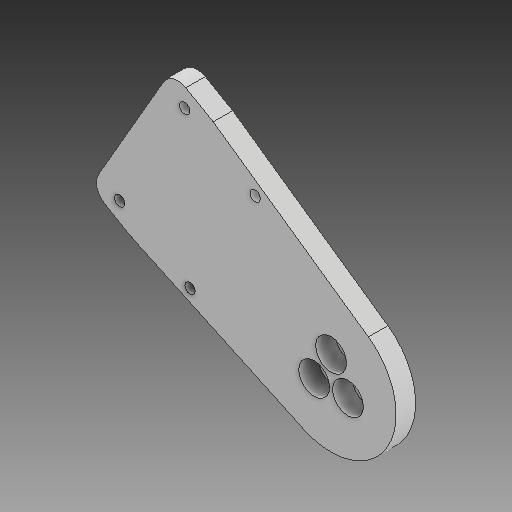
# Autodesk Inventor part: Кронштейн_разлив
Saved by Autodesk Inventor 2022 (Build 260153000, 153)
## iProperties
Created: 2025-01-18
Part Number: Кронштейн_разлив
Material: Типовые
Document SubType Name: Modeling
Designer: Ivan
Density: 1 g/cm^3
Appearance: По умолчанию
Mass: 21.8747 g
Surface Area: 95.7591 cm^2
Volume: 21.8747 cm^3
Author: Ivan
Title: Кронштейн_разлив
Autodesk Inventor part; units mm, degrees
ref_plane "YZ Plane" through (0, 0, 0) normal (1, 0, 0) x (0, 1, 0)
ref_plane "XZ Plane" through (0, 0, 0) normal (0, 1, 0) x (-1, 0, 0)
ref_plane "РабПлоскость1" through (0, -183.0039, -21) normal (0, 0, -1) x (-1, 0, 0)
sketch "Эскиз1" plane through (0, -183.0039, -21) normal (0, 0, -1) x (-1, 0, 0)
  circle A0 centre (-113.4086, 91.5744) radius 1.6 construction
  circle A1 centre (-135.0593, 104.0744) radius 1.6 construction
  circle A2 centre (-155.0593, 69.4334) radius 1.6 construction
  circle A3 centre (-133.4086, 56.9334) radius 1.6 construction
  circle A4 centre (113.4086, 91.5744) radius 1.6 projected
  circle A5 centre (133.4086, 56.9334) radius 1.6 projected
  circle A6 centre (155.0593, 69.4334) radius 1.6 projected
  circle A7 centre (135.0593, 104.0744) radius 1.6 projected
  circle A8 centre (-39.6673, 36.2982) radius 1.6 construction
  circle A9 centre (-64.2558, 29.7097) radius 1.6 construction
  circle A10 centre (55.2558, 45.2982) radius 1.6 construction
  circle A11 centre (48.6673, 20.7097) radius 1.6 construction
  circle A12 centre (-9, -65.9961) radius 1.6 construction
  circle A13 centre (9, -47.9961) radius 1.6 construction
  circle A14 centre (-9, -47.9961) radius 1.6 construction
  circle A15 centre (9, -65.9961) radius 1.6 construction
  circle A16 centre (39.6673, 36.2982) radius 1.6 construction
  circle A17 centre (64.2558, 29.7097) radius 1.6 construction
  circle A18 centre (-55.2558, 45.2982) radius 1.6 construction
  circle A19 centre (-48.6673, 20.7097) radius 1.6 construction
  circle A20 centre (15.6458, -34.8967) radius 0.75 construction
  circle A21 centre (58.9471, -59.8967) radius 0.75 construction
  circle A22 centre (83.9471, -16.5954) radius 0.75 construction
  circle A23 centre (40.6458, 8.4046) radius 0.75 construction
  circle A24 centre (-40.6458, 8.4046) radius 0.75 construction
  circle A25 centre (-83.9471, -16.5954) radius 0.75 construction
  circle A26 centre (-58.9471, -59.8967) radius 0.75 construction
  circle A27 centre (-15.6458, -34.8967) radius 0.75 construction
  circle A28 centre (25, 35.5039) radius 0.75 construction
  circle A29 centre (-25, 35.5039) radius 0.75 construction
  circle A30 centre (-25, 85.5039) radius 0.75 construction
  circle A31 centre (25, 85.5039) radius 0.75 construction
  line L0 (-99.4987, -146.9961) -> (-58.2292, -146.9961) construction
  arc A32 (-58.2292, -146.9961) -> (-50.2665, -135.1021) centre (-78.4573, -124.8415) ccw construction
  line L1 (-50.2665, -135.1021) -> (-34.4151, -91.5508) construction
  arc A33 (-4.446, -71.8642) -> (-34.4151, -91.5508) centre (-6.2243, -101.8114) ccw construction
  arc A34 (-4.446, -71.8642) -> (4.446, -71.8642) centre (0, 3.0039) ccw construction
  arc A35 (34.4151, -91.5508) -> (4.446, -71.8642) centre (6.2243, -101.8114) ccw construction
  line L2 (34.4151, -91.5508) -> (50.2665, -135.1021) construction
  arc A36 (50.2665, -135.1021) -> (58.2292, -146.9961) centre (78.4573, -124.8415) ccw construction
  line L3 (58.2292, -146.9961) -> (99.4987, -146.9961) construction
  arc A37 (99.4987, -146.9961) -> (103.9106, -143.9743) centre (0, 3.0039) ccw construction
  arc A38 (103.9106, -143.9743) -> (113.7491, -106.7304) centre (86.5921, -119.4779) ccw construction
  arc A39 (151.9073, -40.6385) -> (113.7491, -106.7304) centre (155.8424, -86.9717) ccw construction
  arc A40 (151.9073, -40.6385) -> (179.2421, -13.4962) centre (149.3685, -10.7461) ccw construction
  arc A41 (179.2421, -13.4962) -> (99.4987, 153.0039) centre (0, 3.0039) ccw construction
  line L4 (99.4987, 153.0039) -> (78.6769, 153.0039) construction
  line L5 (78.6769, 153.0039) -> (88.1693, 146.3572) construction
  line L6 (88.1693, 146.3572) -> (84.7279, 141.4423) construction
  line L7 (84.7279, 141.4423) -> (72.4406, 150.046) construction
  line L8 (72.4406, 150.046) -> (74.5118, 153.0039) construction
  line L9 (74.5118, 153.0039) -> (65.3792, 153.0039) construction
  line L10 (65.3792, 153.0039) -> (62.0876, 145.0572) construction
  line L11 (62.0876, 145.0572) -> (56.5443, 147.3533) construction
  line L12 (56.5443, 147.3533) -> (58.8849, 153.0039) construction
  line L13 (58.8849, 153.0039) -> (35.5692, 153.0039) construction
  arc A42 (-35.5692, 153.0039) -> (35.5692, 153.0039) centre (0, 182.9552) ccw construction
  line L14 (-35.5692, 153.0039) -> (-58.8849, 153.0039) construction
  line L15 (-58.8849, 153.0039) -> (-56.5443, 147.3533) construction
  line L16 (-56.5443, 147.3533) -> (-62.0876, 145.0572) construction
  line L17 (-62.0876, 145.0572) -> (-65.3792, 153.0039) construction
  line L18 (-65.3792, 153.0039) -> (-74.5118, 153.0039) construction
  line L19 (-74.5118, 153.0039) -> (-72.4406, 150.046) construction
  line L20 (-72.4406, 150.046) -> (-84.7279, 141.4423) construction
  line L21 (-84.7279, 141.4423) -> (-88.1693, 146.3572) construction
  line L22 (-88.1693, 146.3572) -> (-78.6769, 153.0039) construction
  line L23 (-78.6769, 153.0039) -> (-99.4987, 153.0039) construction
  arc A43 (-99.4987, 153.0039) -> (-179.2421, -13.4962) centre (0, 3.0039) ccw construction
  arc A44 (-179.2421, -13.4962) -> (-151.9073, -40.6385) centre (-149.3685, -10.7461) ccw construction
  arc A45 (-113.7491, -106.7304) -> (-151.9073, -40.6385) centre (-155.8424, -86.9717) ccw construction
  arc A46 (-113.7491, -106.7304) -> (-103.9106, -143.9743) centre (-86.5921, -119.4779) ccw construction
  arc A47 (-103.9106, -143.9743) -> (-99.4987, -146.9961) centre (0, 3.0039) ccw construction
  line L24 (-44, 63.0039) -> (-44, 78.0039) construction
  line L25 (-44, 78.0039) -> (-35, 78.0039) construction
  line L26 (-35, 78.0039) -> (-35, 63.0039) construction
  line L27 (-35, 63.0039) -> (-44, 63.0039) construction
  line L28 (-44, 123.0039) -> (-44, 138.0039) construction
  line L29 (-44, 138.0039) -> (-35, 138.0039) construction
  line L30 (-35, 138.0039) -> (-35, 123.0039) construction
  line L31 (-35, 123.0039) -> (-44, 123.0039) construction
  line L32 (44, 108.0039) -> (44, 93.0039) construction
  line L33 (44, 93.0039) -> (35, 93.0039) construction
  line L34 (35, 93.0039) -> (35, 108.0039) construction
  line L35 (35, 108.0039) -> (44, 108.0039) construction
  line L36 (44, 123.0039) -> (35, 123.0039) construction
  line L37 (35, 123.0039) -> (35, 138.0039) construction
  line L38 (35, 138.0039) -> (44, 138.0039) construction
  line L39 (44, 138.0039) -> (44, 123.0039) construction
  line L40 (-35, 93.0039) -> (-44, 93.0039) construction
  line L41 (-44, 93.0039) -> (-44, 108.0039) construction
  line L42 (-44, 108.0039) -> (-35, 108.0039) construction
  line L43 (-35, 108.0039) -> (-35, 93.0039) construction
  line L44 (-15, 119.0039) -> (15, 119.0039) construction
  line L45 (15, 119.0039) -> (15, 113.0039) construction
  line L46 (15, 113.0039) -> (-15, 113.0039) construction
  line L47 (-15, 113.0039) -> (-15, 119.0039) construction
  line L48 (44, 78.0039) -> (44, 63.0039) construction
  line L49 (44, 63.0039) -> (35, 63.0039) construction
  line L50 (35, 63.0039) -> (35, 78.0039) construction
  line L51 (35, 78.0039) -> (44, 78.0039) construction
  line L52 (73.9615, 11.1091) -> (86.9519, 3.6091) construction
  line L53 (86.9519, 3.6091) -> (82.4519, -4.1852) construction
  line L54 (82.4519, -4.1852) -> (69.4615, 3.3148) construction
  line L55 (69.4615, 3.3148) -> (73.9615, 11.1091) construction
  line L56 (125.923, -18.8909) -> (138.9134, -26.3909) construction
  line L57 (138.9134, -26.3909) -> (134.4134, -34.1852) construction
  line L58 (134.4134, -34.1852) -> (121.423, -26.6852) construction
  line L59 (121.423, -26.6852) -> (125.923, -18.8909) construction
  line L60 (68.9327, -87.6012) -> (55.9423, -80.1012) construction
  line L61 (55.9423, -80.1012) -> (60.4423, -72.307) construction
  line L62 (60.4423, -72.307) -> (73.4327, -79.807) construction
  line L63 (73.4327, -79.807) -> (68.9327, -87.6012) construction
  line L64 (81.923, -95.1012) -> (86.423, -87.307) construction
  line L65 (86.423, -87.307) -> (99.4134, -94.807) construction
  line L66 (99.4134, -94.807) -> (94.9134, -102.6012) construction
  line L67 (94.9134, -102.6012) -> (81.923, -95.1012) construction
  line L68 (95.4423, -11.6852) -> (99.9423, -3.8909) construction
  line L69 (99.9423, -3.8909) -> (112.9327, -11.3909) construction
  line L70 (112.9327, -11.3909) -> (108.4327, -19.1852) construction
  line L71 (108.4327, -19.1852) -> (95.4423, -11.6852) construction
  line L72 (107.9589, -42.0057) -> (92.9589, -67.9864) construction
  line L73 (92.9589, -67.9864) -> (87.7628, -64.9864) construction
  line L74 (87.7628, -64.9864) -> (102.7628, -39.0057) construction
  line L75 (102.7628, -39.0057) -> (107.9589, -42.0057) construction
  line L76 (42.9519, -72.6012) -> (29.9615, -65.1012) construction
  line L77 (29.9615, -65.1012) -> (34.4615, -57.307) construction
  line L78 (34.4615, -57.307) -> (47.4519, -64.807) construction
  line L79 (47.4519, -64.807) -> (42.9519, -72.6012) construction
  line L80 (-47.4519, -64.807) -> (-34.4615, -57.307) construction
  line L81 (-34.4615, -57.307) -> (-29.9615, -65.1012) construction
  line L82 (-29.9615, -65.1012) -> (-42.9519, -72.6012) construction
  line L83 (-42.9519, -72.6012) -> (-47.4519, -64.807) construction
  line L84 (-82.4519, -4.1852) -> (-86.9519, 3.6091) construction
  line L85 (-86.9519, 3.6091) -> (-73.9615, 11.1091) construction
  line L86 (-73.9615, 11.1091) -> (-69.4615, 3.3148) construction
  line L87 (-69.4615, 3.3148) -> (-82.4519, -4.1852) construction
  line L88 (-102.7628, -39.0057) -> (-87.7628, -64.9864) construction
  line L89 (-87.7628, -64.9864) -> (-92.9589, -67.9864) construction
  line L90 (-92.9589, -67.9864) -> (-107.9589, -42.0057) construction
  line L91 (-107.9589, -42.0057) -> (-102.7628, -39.0057) construction
  line L92 (-73.4327, -79.807) -> (-60.4423, -72.307) construction
  line L93 (-60.4423, -72.307) -> (-55.9423, -80.1012) construction
  line L94 (-55.9423, -80.1012) -> (-68.9327, -87.6012) construction
  line L95 (-68.9327, -87.6012) -> (-73.4327, -79.807) construction
  line L96 (-134.4134, -34.1852) -> (-138.9134, -26.3909) construction
  line L97 (-138.9134, -26.3909) -> (-125.923, -18.8909) construction
  line L98 (-125.923, -18.8909) -> (-121.423, -26.6852) construction
  line L99 (-121.423, -26.6852) -> (-134.4134, -34.1852) construction
  line L100 (-108.4327, -19.1852) -> (-112.9327, -11.3909) construction
  line L101 (-112.9327, -11.3909) -> (-99.9423, -3.8909) construction
  line L102 (-99.9423, -3.8909) -> (-95.4423, -11.6852) construction
  line L103 (-95.4423, -11.6852) -> (-108.4327, -19.1852) construction
  line L104 (-99.4134, -94.807) -> (-86.423, -87.307) construction
  line L105 (-86.423, -87.307) -> (-81.923, -95.1012) construction
  line L106 (-81.923, -95.1012) -> (-94.9134, -102.6012) construction
  line L107 (-94.9134, -102.6012) -> (-99.4134, -94.807) construction
  line L108 (-113.3982, 121.3672) -> (-116.8396, 126.2821) construction
  line L109 (-116.8396, 126.2821) -> (-104.5524, 134.8857) construction
  line L110 (-104.5524, 134.8857) -> (-101.1109, 129.9708) construction
  line L111 (-101.1109, 129.9708) -> (-113.3982, 121.3672) construction
  line L112 (-162.2551, 7.1612) -> (-163.5624, -7.7817) construction
  line L113 (-163.5624, -7.7817) -> (-169.5396, -7.2588) construction
  line L114 (-169.5396, -7.2588) -> (-168.2323, 7.6842) construction
  line L115 (-168.2323, 7.6842) -> (-162.2551, 7.1612) construction
  line L116 (-119.365, -9.6849) -> (-118.5818, -15.6335) construction
  line L117 (-118.5818, -15.6335) -> (-133.4535, -17.5914) construction
  line L118 (-133.4535, -17.5914) -> (-134.2366, -11.6428) construction
  line L119 (-134.2366, -11.6428) -> (-119.365, -9.6849) construction
  line L120 (-73.1685, -110.4878) -> (-65.3227, -97.7033) construction
  line L121 (-65.3227, -97.7033) -> (-60.2089, -100.8416) construction
  line L122 (-60.2089, -100.8416) -> (-68.0546, -113.6261) construction
  line L123 (-68.0546, -113.6261) -> (-73.1685, -110.4878) construction
  line L124 (-165.1818, 42.551) -> (-159.2046, 42.028) construction
  line L125 (-159.2046, 42.028) -> (-160.512, 27.0851) construction
  line L126 (-160.512, 27.0851) -> (-166.4892, 27.608) construction
  line L127 (-166.4892, 27.608) -> (-165.1818, 42.551) construction
  line L128 (-153.2824, -20.202) -> (-168.154, -22.1599) construction
  line L129 (-168.154, -22.1599) -> (-168.9372, -16.2112) construction
  line L130 (-168.9372, -16.2112) -> (-154.0655, -14.2533) construction
  line L131 (-154.0655, -14.2533) -> (-153.2824, -20.202) construction
  line L132 (-86.3613, -143.4567) -> (-91.4751, -140.3184) construction
  line L133 (-91.4751, -140.3184) -> (-83.6294, -127.5339) construction
  line L134 (-83.6294, -127.5339) -> (-78.5156, -130.6722) construction
  line L135 (-78.5156, -130.6722) -> (-86.3613, -143.4567) construction
  line L136 (-48.8906, 128.8757) -> (-43.1504, 115.0175) construction
  line L137 (-43.1504, 115.0175) -> (-48.6937, 112.7214) construction
  line L138 (-48.6937, 112.7214) -> (-54.4339, 126.5796) construction
  line L139 (-54.4339, 126.5796) -> (-48.8906, 128.8757) construction
  line L140 (101.1109, 129.9708) -> (104.5524, 134.8857) construction
  line L141 (104.5524, 134.8857) -> (116.8396, 126.2821) construction
  line L142 (116.8396, 126.2821) -> (113.3982, 121.3672) construction
  line L143 (113.3982, 121.3672) -> (101.1109, 129.9708) construction
  line L144 (48.8906, 128.8757) -> (54.4339, 126.5796) construction
  line L145 (54.4339, 126.5796) -> (48.6937, 112.7214) construction
  line L146 (48.6937, 112.7214) -> (43.1504, 115.0175) construction
  line L147 (43.1504, 115.0175) -> (48.8906, 128.8757) construction
  line L148 (78.5156, -130.6722) -> (83.6294, -127.5339) construction
  line L149 (83.6294, -127.5339) -> (91.4751, -140.3184) construction
  line L150 (91.4751, -140.3184) -> (86.3613, -143.4567) construction
  line L151 (86.3613, -143.4567) -> (78.5156, -130.6722) construction
  line L152 (153.2824, -20.202) -> (154.0655, -14.2533) construction
  line L153 (154.0655, -14.2533) -> (168.9372, -16.2112) construction
  line L154 (168.9372, -16.2112) -> (168.154, -22.1599) construction
  line L155 (168.154, -22.1599) -> (153.2824, -20.202) construction
  line L156 (166.4892, 27.608) -> (160.512, 27.0851) construction
  line L157 (160.512, 27.0851) -> (159.2046, 42.028) construction
  line L158 (159.2046, 42.028) -> (165.1818, 42.551) construction
  line L159 (165.1818, 42.551) -> (166.4892, 27.608) construction
  line L160 (73.1685, -110.4878) -> (68.0546, -113.6261) construction
  line L161 (68.0546, -113.6261) -> (60.2089, -100.8416) construction
  line L162 (60.2089, -100.8416) -> (65.3227, -97.7033) construction
  line L163 (65.3227, -97.7033) -> (73.1685, -110.4878) construction
  line L164 (134.2366, -11.6428) -> (133.4535, -17.5914) construction
  line L165 (133.4535, -17.5914) -> (118.5818, -15.6335) construction
  line L166 (118.5818, -15.6335) -> (119.365, -9.6849) construction
  line L167 (119.365, -9.6849) -> (134.2366, -11.6428) construction
  line L168 (162.2551, 7.1612) -> (168.2323, 7.6842) construction
  line L169 (168.2323, 7.6842) -> (169.5396, -7.2588) construction
  line L170 (169.5396, -7.2588) -> (163.5624, -7.7817) construction
  line L171 (163.5624, -7.7817) -> (162.2551, 7.1612) construction
  arc A48 (3.25, -9.7608) -> (3.5417, -10.4667) centre (4.25, -9.7608) ccw construction
  arc A49 (-3.5417, -10.4667) -> (3.5417, -10.4667) centre (0, -13.9961) ccw construction
  arc A50 (-3.5417, -10.4667) -> (-3.25, -9.7608) centre (-4.25, -9.7608) ccw construction
  line L172 (-3.25, -9.7608) -> (-3.25, -8.2183) construction
  arc A51 (-3.25, -8.2183) -> (-3.8958, -7.2831) centre (-4.25, -8.2183) ccw construction
  arc A52 (-8.4764, -4.0069) -> (-3.8958, -7.2831) centre (0, 3.0039) ccw construction
  arc A53 (-8.4764, -4.0069) -> (-9.747, -3.7782) centre (-9.247, -4.6442) ccw construction
  line L173 (-9.747, -3.7782) -> (-10.7583, -4.3621) construction
  arc A54 (-10.7583, -4.3621) -> (-11.1244, -5.7281) centre (-10.2583, -5.2281) ccw construction
  line L174 (-11.1244, -5.7281) -> (-9.6244, -8.3262) construction
  line L175 (-9.6244, -8.3262) -> (-11.3564, -9.3262) construction
  line L176 (-11.3564, -9.3262) -> (-16.3564, -0.6659) construction
  line L177 (-16.3564, -0.6659) -> (-14.6244, 0.3341) construction
  line L178 (-14.6244, 0.3341) -> (-13.1244, -2.264) construction
  arc A55 (-13.1244, -2.264) -> (-11.7583, -2.63) centre (-12.2583, -1.764) ccw construction
  line L179 (-11.7583, -2.63) -> (-10.747, -2.0461) construction
  arc A56 (-10.747, -2.0461) -> (-10.3097, -0.8314) centre (-11.247, -1.1801) ccw construction
  arc A57 (-10.8567, 4.7735) -> (-10.3097, -0.8314) centre (0, 3.0039) ccw construction
  arc A58 (-10.8567, 4.7735) -> (-11.3437, 5.8004) centre (-11.8437, 4.9344) ccw construction
  line L180 (-11.3437, 5.8004) -> (-12.6796, 6.5717) construction
  arc A59 (-12.6796, 6.5717) -> (-13.4367, 6.6721) centre (-13.1796, 5.7057) ccw construction
  arc A60 (-9.8951, 12.8064) -> (-13.4367, 6.6721) centre (-14.7224, 11.5039) ccw construction
  arc A61 (-9.8951, 12.8064) -> (-9.4296, 12.2009) centre (-8.9296, 13.0669) ccw construction
  line L181 (-9.4296, 12.2009) -> (-8.0937, 11.4296) construction
  arc A62 (-8.0937, 11.4296) -> (-6.9609, 11.5213) centre (-7.5937, 12.2956) ccw construction
  arc A63 (-1.8333, 13.8501) -> (-6.9609, 11.5213) centre (0, 3.0039) ccw construction
  arc A64 (-1.8333, 13.8501) -> (-1, 14.8361) centre (-2, 14.8361) ccw construction
  line L182 (-1, 14.8361) -> (-1, 16.0039) construction
  arc A65 (-1, 16.0039) -> (-2, 17.0039) centre (-2, 16.0039) ccw construction
  line L183 (-2, 17.0039) -> (-5, 17.0039) construction
  line L184 (-5, 17.0039) -> (-5, 19.0039) construction
  line L185 (-5, 19.0039) -> (5, 19.0039) construction
  line L186 (5, 19.0039) -> (5, 17.0039) construction
  line L187 (5, 17.0039) -> (2, 17.0039) construction
  arc A66 (2, 17.0039) -> (1, 16.0039) centre (2, 16.0039) ccw construction
  line L188 (1, 16.0039) -> (1, 14.8361) construction
  arc A67 (1, 14.8361) -> (1.8333, 13.8501) centre (2, 14.8361) ccw construction
  arc A68 (6.9609, 11.5213) -> (1.8333, 13.8501) centre (0, 3.0039) ccw construction
  arc A69 (6.9609, 11.5213) -> (8.0937, 11.4296) centre (7.5937, 12.2956) ccw construction
  line L189 (8.0937, 11.4296) -> (9.4296, 12.2009) construction
  arc A70 (9.4296, 12.2009) -> (9.8951, 12.8064) centre (8.9296, 13.0669) ccw construction
  arc A71 (13.4367, 6.6721) -> (9.8951, 12.8064) centre (14.7224, 11.5039) ccw construction
  arc A72 (13.4367, 6.6721) -> (12.6796, 6.5717) centre (13.1796, 5.7057) ccw construction
  line L190 (12.6796, 6.5717) -> (11.3437, 5.8004) construction
  arc A73 (11.3437, 5.8004) -> (10.8567, 4.7735) centre (11.8437, 4.9344) ccw construction
  arc A74 (10.3097, -0.8314) -> (10.8567, 4.7735) centre (0, 3.0039) ccw construction
  arc A75 (10.3097, -0.8314) -> (10.747, -2.0461) centre (11.247, -1.1801) ccw construction
  line L191 (10.747, -2.0461) -> (11.7583, -2.63) construction
  arc A76 (11.7583, -2.63) -> (13.1244, -2.264) centre (12.2583, -1.764) ccw construction
  line L192 (13.1244, -2.264) -> (14.6244, 0.3341) construction
  line L193 (14.6244, 0.3341) -> (16.3564, -0.6659) construction
  line L194 (16.3564, -0.6659) -> (11.3564, -9.3262) construction
  line L195 (11.3564, -9.3262) -> (9.6244, -8.3262) construction
  line L196 (9.6244, -8.3262) -> (11.1244, -5.7281) construction
  arc A77 (11.1244, -5.7281) -> (10.7583, -4.3621) centre (10.2583, -5.2281) ccw construction
  line L197 (10.7583, -4.3621) -> (9.747, -3.7782) construction
  arc A78 (9.747, -3.7782) -> (8.4764, -4.0069) centre (9.247, -4.6442) ccw construction
  arc A79 (3.8958, -7.2831) -> (8.4764, -4.0069) centre (0, 3.0039) ccw construction
  arc A80 (3.8958, -7.2831) -> (3.25, -8.2183) centre (4.25, -8.2183) ccw construction
  line L198 (3.25, -8.2183) -> (3.25, -9.7608) construction
  arc A81 (-54.1242, 54.9228) -> (-95.9802, 95.0735) centre (-75.0522, 74.9982) ccw construction
  arc A82 (-54.1242, 54.9228) -> (-72.0252, 23.9174) centre (0, 3.0039) ccw construction
  arc A83 (-127.7247, 40.0905) -> (-72.0252, 23.9174) centre (-99.8749, 32.0039) ccw construction
  arc A84 (-95.9802, 95.0735) -> (-127.7247, 40.0905) centre (0, 3.0039) ccw construction
  arc A85 (72.0252, 23.9174) -> (127.7247, 40.0905) centre (99.8749, 32.0039) ccw construction
  arc A86 (72.0252, 23.9174) -> (54.1242, 54.9228) centre (0, 3.0039) ccw construction
  arc A87 (95.9802, 95.0735) -> (54.1242, 54.9228) centre (75.0522, 74.9982) ccw construction
  arc A88 (127.7247, 40.0905) -> (95.9802, 95.0735) centre (0, 3.0039) ccw construction
  circle A89 centre (88.6033, 57.4599) radius 21.579 construction
  circle A90 centre (0, 3.0039) radius 104 construction
  line L199 (0, 3.0039) -> (115.1814, 69.5039) construction
  line L200 (139.0544, 112.1546) -> (164.0544, 68.8533)
  line L201 (164.0544, 68.8533) -> (151.304, 61.4918)
  line L202 (151.304, 61.4918) -> (98.519, 36.8778)
  arc A91 (72.7461, 45.0039) -> (98.519, 36.8778) centre (90.0666, 55.0039) ccw
  line L203 (139.0544, 112.1546) -> (126.304, 104.7931)
  line L204 (126.304, 104.7931) -> (78.5951, 71.387)
  arc A92 (78.5951, 71.387) -> (72.7461, 45.0039) centre (90.0666, 55.0039) ccw
  circle A93 centre (90.0666, 55.0039) radius 6 construction
  circle A94 centre (84.8705, 52.0039) radius 4.75
  circle A95 centre (95.2628, 52.0039) radius 4.75
  circle A96 centre (90.0666, 61.0039) radius 4.75
  point P0 (0, 183.0039)
  dimension "d5" = 12
  dimension "d0" = 25
  dimension "d1" = 175
  dimension "d2" = 5
  dimension "d3" = 20
  dimension "d4" = 9.5
  dimension "d8" = 360
  constraints: 12 end point, 7 point on circle, 6 centre point, 3 symmetric about line, 2 coincident, 2 perpendicular, 2 point on line, 1 line through centre, 1 tangent, 11 other
  measures "d0" distance between parallel lines of L201 L199
  measures "d1" distance from line of A47.centre L200
  measures "d2" angle of L201 L202
  measures "d3" radius of A91
  measures "d4" diameter of A94
extrude "Выдавливание1" add sketch "Эскиз1" along normal blind 6
fillet "Сопряжение1" radius 5 2 edges at (-164.0544, -114.1506, -24) (-139.0544, -70.8494, -24)
